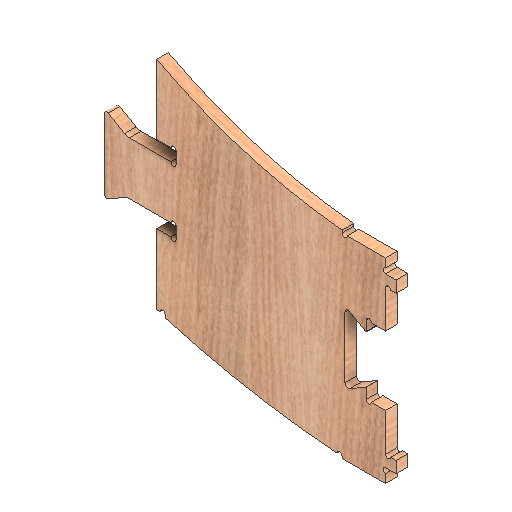
# Autodesk Inventor part: Support D
Saved by Autodesk Inventor 2021 (Build 250183000, 183)
## iProperties
Created: 2020-05-09
Part Number: Support D
Material: Wood (Birch)
Document SubType Name: Modeling
Designer: Dan Wikman
Density: 0.55 g/cm^3
Appearance: Birch - Natural Polished
Mass: 1108.47 g
Surface Area: 2597.85 cm^2
Volume: 2015.41 cm^3
Autodesk Inventor part; units mm, degrees
ref_plane "YZ Plane" through (0, 0, 0) normal (1, 0, 0) x (0, 1, 0)
ref_plane "XZ Plane" through (0, 0, 0) normal (0, 1, 0) x (-1, 0, 0)
ref_plane "XY Plane" through (0, 0, 0) normal (0, 0, 1) x (1, 0, 0)
sketch "CONTOURS" plane through (0, 0, 0) normal (0, 0, 1) x (1, 0, 0)
  line L0 (2304.856, 1106.9778) -> (2304.856, 1110.7555)
  arc A0 (2016.715, 1196.7237) -> (2304.856, 1110.7555) centre (2382.3562, 1896.3821) ccw
  line L1 (2016.715, 1196.7237) -> (2016.715, 1088.6982)
  line L2 (2016.715, 1088.6982) -> (2038.715, 1088.6982)
  arc A1 (2046.715, 1088.6982) -> (2038.715, 1088.6982) centre (2042.715, 1088.6982) ccw
  line L3 (2046.715, 1088.6982) -> (2046.715, 1069.6982)
  arc A2 (2038.715, 1069.6982) -> (2046.715, 1069.6982) centre (2042.715, 1069.6982) ccw
  line L4 (2038.715, 1069.6982) -> (2015.215, 1069.6982)
  line L5 (2015.215, 1069.6982) -> (1974.2342, 1069.6982)
  arc A3 (1966.7342, 1071.7078) -> (1974.2342, 1069.6982) centre (1974.2342, 1084.6982) ccw
  line L6 (1966.7342, 1071.7078) -> (1941.215, 1086.4414)
  arc A4 (1941.215, 1086.4414) -> (1935.215, 1082.9773) centre (1939.215, 1082.9773) ccw
  line L7 (1935.215, 1082.9773) -> (1935.215, 974.4192)
  arc A5 (1935.215, 974.4192) -> (1941.215, 970.9551) centre (1939.215, 974.4192) ccw
  line L8 (1941.215, 970.9551) -> (1966.7342, 985.6886)
  arc A6 (1974.2342, 987.6982) -> (1966.7342, 985.6886) centre (1974.2342, 972.6982) ccw
  line L9 (1974.2342, 987.6982) -> (2015.215, 987.6982)
  line L10 (2015.215, 987.6982) -> (2038.715, 987.6982)
  arc A7 (2046.715, 987.6982) -> (2038.715, 987.6982) centre (2042.715, 987.6982) ccw
  line L11 (2046.715, 987.6982) -> (2046.715, 968.6982)
  arc A8 (2038.715, 968.6982) -> (2046.715, 968.6982) centre (2042.715, 968.6982) ccw
  line L12 (2038.715, 968.6982) -> (2016.715, 968.6982)
  line L13 (2016.715, 968.6982) -> (2016.715, 859.6983)
  line L14 (2016.715, 859.6983) -> (2021.856, 859.6983)
  arc A9 (2029.856, 859.6983) -> (2021.856, 859.6983) centre (2025.856, 859.6983) ccw
  line L15 (2029.856, 859.6983) -> (2029.856, 855.0959)
  arc A10 (2029.856, 855.0959) -> (2296.8765, 806.6253) centre (2393.477, 2098.5207) ccw
  arc A11 (2304.856, 806.0534) -> (2296.8765, 806.6253) centre (2300.8659, 806.3333) ccw
  line L16 (2304.856, 806.0534) -> (2304.856, 803.3051)
  line L17 (2304.856, 803.3051) -> (2372.356, 803.3051)
  line L18 (2372.356, 803.3051) -> (2372.356, 816.6401)
  arc A12 (2372.356, 824.6401) -> (2372.356, 816.6401) centre (2372.356, 820.6401) ccw
  line L19 (2372.356, 824.6401) -> (2388.856, 824.6401)
  line L20 (2388.856, 824.6401) -> (2388.856, 842.6401)
  line L21 (2388.856, 842.6401) -> (2380.356, 842.6401)
  arc A13 (2372.356, 842.6401) -> (2380.356, 842.6401) centre (2376.356, 842.6401) ccw
  line L22 (2372.356, 842.6401) -> (2372.356, 901.6415)
  line L23 (2372.356, 901.6415) -> (2350.356, 901.6415)
  arc A14 (2342.356, 901.6415) -> (2350.356, 901.6415) centre (2346.356, 901.6415) ccw
  line L24 (2342.356, 901.6415) -> (2342.356, 918.031)
  line L25 (2342.356, 918.031) -> (2342.1144, 917.9007)
  line L26 (2342.1144, 917.9007) -> (2341.8753, 917.7658)
  line L27 (2341.8753, 917.7658) -> (2316.715, 903.2395)
  arc A15 (2309.215, 907.5697) -> (2316.715, 903.2395) centre (2314.215, 907.5697) ccw
  line L28 (2309.215, 907.5697) -> (2309.215, 1002.7133)
  arc A16 (2316.715, 1007.0434) -> (2309.215, 1002.7133) centre (2314.215, 1002.7133) ccw
  line L29 (2316.715, 1007.0434) -> (2341.8753, 992.5171)
  line L30 (2341.8753, 992.5171) -> (2342.1144, 992.3822)
  line L31 (2342.1144, 992.3822) -> (2342.356, 992.252)
  line L32 (2342.356, 992.252) -> (2342.356, 1008.6415)
  arc A17 (2350.356, 1008.6415) -> (2342.356, 1008.6415) centre (2346.356, 1008.6415) ccw
  line L33 (2350.356, 1008.6415) -> (2372.356, 1008.6415)
  line L34 (2372.356, 1008.6415) -> (2372.356, 1067.6428)
  arc A18 (2380.356, 1067.6428) -> (2372.356, 1067.6428) centre (2376.356, 1067.6428) ccw
  line L35 (2380.356, 1067.6428) -> (2388.856, 1067.6428)
  line L36 (2388.856, 1067.6428) -> (2388.856, 1085.6428)
  line L37 (2388.856, 1085.6428) -> (2372.356, 1085.6428)
  arc A19 (2372.356, 1093.6428) -> (2372.356, 1085.6428) centre (2372.356, 1089.6428) ccw
  line L38 (2372.356, 1093.6428) -> (2372.356, 1106.9778)
  line L39 (2372.356, 1106.9778) -> (2312.856, 1106.9778)
  arc A20 (2304.856, 1106.9778) -> (2312.856, 1106.9778) centre (2308.856, 1106.9778) ccw
  constraints: 80 end point, 42 point on circle, 21 centre point
sketch "LETTERS" plane through (0, 0, 0) normal (0, 0, 1) x (1, 0, 0)
  line L0 (2156.0965, 986.9239) -> (2156.0965, 980.0933)
  line L1 (2156.0965, 980.0933) -> (2175.9213, 980.0933)
  line L2 (2175.9213, 980.0933) -> (2175.9213, 986.9239)
  arc A0 (2175.9213, 986.9239) -> (2156.0965, 986.9239) centre (2166.0089, 986.9239) ccw
  constraints: 6 end point, 2 point on circle, 2 tangent, 1 centre point, 1 parallel, 1 perpendicular
extrude "Extrusion4" add sketch "CONTOURS" along normal blind 18
body "Solid1"
